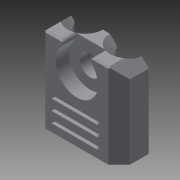
# Autodesk Inventor part: key_half_screw
Saved by Autodesk Inventor 2014 (Build 180170000, 170)
## iProperties
Created: 2014-05-24
Part Number: key_half_screw
Material: Generic
Document SubType Name: Modeling
Designer: brent
Density: 1 g/cm^3
Appearance: Default
Author: brent
Autodesk Inventor part; units mm, degrees
ref_plane "YZ Plane" through (0, 0, 0) normal (1, 0, 0) x (0, 1, 0)
ref_plane "XZ Plane" through (0, 0, 0) normal (0, 1, 0) x (-1, 0, 0)
ref_plane "XY Plane" through (0, 0, 0) normal (0, 0, 1) x (1, 0, 0)
sketch "Sketch1" plane through (0, 0, 0) normal (0, 1, 0) x (-1, 0, 0)
  line L0 (-10.2591, 9.049) -> (9.7409, 9.049)
  line L1 (9.7409, 9.049) -> (9.7409, -10.951)
  line L2 (9.7409, -10.951) -> (-10.2591, -10.951)
  line L3 (-10.2591, -10.951) -> (-10.2591, 9.049)
  point P0 (0, 0)
  dimension "d0" = 20
  dimension "d1" = 20
  constraints: 8 end point, 2 parallel, 1 horizontal, 1 perpendicular
  measures "d0" distance of L1.end L2.end
  measures "d1" distance of L0.end L1.end
extrude "Extrusion1" add sketch "Sketch1" along normal blind 7
sketch "Sketch2" plane through (-9.7409, 0, 9.049) normal (0, 0, 1) x (1, 0, 0)
  line L0 (20, 0) -> (0, 0) projected
  line L1 (20, 0) -> (20, 7) projected
  line L2 (0, 0) -> (0, 7) projected
  circle A0 centre (15, 0) radius 3.375
  circle A1 centre (5, 0) radius 3.375
  point P0 (9.7409, 0)
  dimension "d4" = 6.75
  dimension "d5" = 6.75
  dimension "d6" = 5
  dimension "d7" = 5
  dimension "d32" = 10
  constraints: 2 centre point, 2 point on line
  measures "d4" diameter of A0
  measures "d5" diameter of A1
  measures "d6" distance from line of A0.centre L1
  measures "d7" distance from line of L2 A1.centre
  measures "d32" distance of A1.centre A0.centre
extrude "Extrusion2" cut sketch "Sketch2" against normal blind 7.4
sketch "Sketch3" plane through (-9.7409, 0, 1.649) normal (0, 0, 1) x (1, 0, 0)
  arc A0 (8.375, 0) -> (1.625, 0) centre (5, 0) ccw projected
  line L0 (18.375, 0) -> (11.625, 0) projected
  arc A1 (18.375, 0) -> (11.625, 0) centre (15, 0) ccw projected
  circle A2 centre (15, 0) radius 2.25
  circle A3 centre (5, 0) radius 2.25
  point P0 (9.7409, 0)
  dimension "d10" = 4.5
  dimension "d11" = 4.5
  constraints: 2 centre point, 2 coincident
  measures "d10" diameter of A2
  measures "d11" diameter of A3
extrude "Extrusion3" cut sketch "Sketch3" against normal through all contours A2 L0 | L0 A2 | A3
sketch "Sketch4" plane through (0, 0, 0) normal (0, -1, 0) x (1, 0, 0)
  line L0 (-2.4909, 1.649) -> (-2.4909, -10.951) projected
  line L1 (3.0091, -10.951) -> (3.0091, 1.649) projected
  circle A0 centre (0.2591, -6.0003) radius 2.4765
  point P0 (0, 0)
  dimension "d14" = 4.953
  dimension "d15" = 5.5
  dimension "d16" = 2.75
  constraints: 1 centre point
  measures "d14" diameter of A0
  measures "d15" distance between parallel lines of L1 L0
  measures "d16" distance from line of A0.centre L1
extrude "Extrusion4" cut sketch "Sketch4" against normal through all
chamfer "Chamfer1" distance 1.905 angle 45 2 edges at (5.2591, 2.25, -10.951) (-4.7409, 2.25, -10.951)
chamfer "Chamfer2" distance 0.381 angle 45 5 edges at (-2.4909, 0, -3.6985) (-6.9909, 0, -3.6985) (7.5091, 0, -3.6985) (3.0091, 0, -3.6985) (0.2591, 7, -10.951)
chamfer "Chamfer3" distance 2.54 angle 45 4 edges at (-9.7409, 7, -0.7605) (10.2591, 7, -0.7605) (-9.7409, 3.3095, -10.951) (10.2591, 3.3095, -10.951)
sketch "Sketch5" plane through (0, 7, 0) normal (0, 1, 0) x (1, 0, 0)
  line L0 (-7.2009, 10.57) -> (7.7191, 10.57) projected
  circle A0 centre (0.2591, 6.0003) radius 2.4765 projected
  line L1 (3.1554, 0.9838) -> (-2.6371, 0.9838)
  line L2 (-2.6371, 0.9838) -> (-5.5334, 6.0003)
  line L3 (-5.5334, 6.0003) -> (-2.6371, 11.0168)
  line L4 (-2.6371, 11.0168) -> (3.1554, 11.0168)
  line L5 (3.1554, 11.0168) -> (6.0517, 6.0003)
  line L6 (6.0517, 6.0003) -> (3.1554, 0.9838)
  circle A1 centre (0.2591, 6.0003) radius 5.0165
  point P0 (0, 0)
  dimension "d29" = 10.033
  dimension "d47" = 10.033
  constraints: 12 end point, 2 coincident, 1 centre point, 1 parallel, 13 other
  measures "d29" distance between parallel lines of L5 L2
  measures "d47" diameter of A1
extrude "Extrusion5" cut sketch "Sketch5" against normal blind 3.175 contours A1 L0 | L0 A1
sketch "Sketch6" plane through (0, 7, 0) normal (0, 1, 0) x (1, 0, 0)
  line L0 (-7.2009, -9.049) -> (-7.2009, 10.57) projected
  line L1 (-7.2009, -9.049) -> (7.7191, -9.049) projected
  line L2 (7.7191, 10.57) -> (7.7191, -9.049) projected
  line L3 (-7.2009, 10.57) -> (7.7191, 10.57) projected
  line L4 (-4.6609, -7.144) -> (5.1791, -7.144) construction
  line L5 (-4.6609, -7.779) -> (5.1791, -7.779)
  line L6 (5.1791, -6.509) -> (-4.6609, -6.509)
  arc A0 (-4.6609, -6.509) -> (-4.6609, -7.779) centre (-4.6609, -7.144) ccw
  arc A1 (5.1791, -7.779) -> (5.1791, -6.509) centre (5.1791, -7.144) ccw
  line L7 (-4.6609, -5.239) -> (5.1791, -5.239)
  line L8 (5.1791, -3.969) -> (-4.6609, -3.969)
  arc A2 (-4.6609, -3.969) -> (-4.6609, -5.239) centre (-4.6609, -4.604) ccw
  arc A3 (5.1791, -5.239) -> (5.1791, -3.969) centre (5.1791, -4.604) ccw
  line L9 (-4.6609, -2.699) -> (5.1791, -2.699)
  line L10 (5.1791, -1.429) -> (-4.6609, -1.429)
  arc A4 (-4.6609, -1.429) -> (-4.6609, -2.699) centre (-4.6609, -2.064) ccw
  arc A5 (5.1791, -2.699) -> (5.1791, -1.429) centre (5.1791, -2.064) ccw
  point P0 (3.4133, 10.57)
  point P1 (0, 0)
  point P2 (0.2591, -7.144)
  dimension "d33" = 1.27
  dimension "d34" = 2.54
  dimension "d35" = 2.54
  dimension "d36" = 1.905
  dimension "d39" = 2.54
  constraints: 16 end point, 12 point on circle, 6 centre point, 4 tangent, 2 parallel, 1 midpoint, 1 vertical, 20 other
  measures "d33" diameter of A1
  measures "d34" distance from line of L2 L4.end
  measures "d35" distance from line of L0 L4.start
  measures "d36" distance from line of L1 point (0.259, -7.144)
  measures "d39" distance of L5.start L7.start
extrude "Extrusion6" add sketch "Sketch6" along normal blind 0.762 contours A0 L6 A1 L5 | A2 L8 A3 L7 | A4 L10 A5 L9
fillet "Fillet1" radius 0.7937 2 edges at (1.0688, 5.222, -10.951) (-0.5505, 5.222, -10.951)
move or copy body "Move Body1" bodies to move or copy 1 copy no rotation origin (0, 0, 0) rotation axis (1, 0, 0) rotation angle 90
equation "\"d16\" = 0.5 * d15"
body "Solid1"
